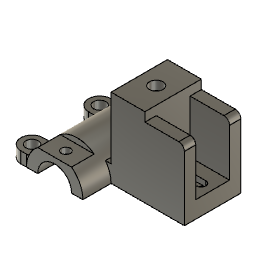
drawing_23 (Autodesk Fusion 360 design; units mm, degrees)
Autodesk Fusion 360 part; units mm, degrees
sketch "Sketch1" plane through (0, 0, 0) normal (0, 0, 1) x (1, 0, 0)
  line L0 (0, 0) -> (-32.5, 0)
  line L1 (-32.5, 0) -> (-32.5, 25)
  line L2 (-32.5, 25) -> (32.5, 25)
  line L3 (32.5, 25) -> (32.5, -25)
  line L4 (32.5, -25) -> (-32.5, -25)
  line L5 (-32.5, -25) -> (-32.5, 25)
  dimension "d1" = 32.5
  dimension "d2" = 25
  dimension "d3" = 65
  dimension "d4" = 50
  constraint coincident L0.start origin
  constraint horizontal L0
  constraint perpendicular L0 L1
  constraint horizontal L2
  constraint vertical L3
  constraint horizontal L4
  constraint vertical L5
  measures "d1" distance of L0.start L0.end
  measures "d2" distance of L0.end L1.end
  measures "d3" distance of L1.end L2.end
  measures "d4" distance of L1.end L4.end
extrude "Extrude1" add sketch "Sketch1" along normal blind 62 makes body 1
sketch "Sketch2" plane through (0, -25, 0) normal (0, -1, 0) x (1, 0, 0)
  line L0 (-32.5, 0) -> (32.5, 0)
  line L1 (32.5, 0) -> (32.5, 62)
  line L2 (32.5, 62) -> (-32.5, 62)
  line L3 (-32.5, 62) -> (-32.5, 0)
  line L4 (32.5, 57) -> (32.5, 36)
  line L5 (27.5, 62) -> (24, 62)
  arc A0 (32.5, 57) -> (27.5, 62) centre (27.5, 57) ccw
  dimension "d7" = 5
  constraint coincident L1 L4.end
  constraint perpendicular L2 L4
  constraint coincident L2 L5.end
  constraint perpendicular L1 L5
  constraint tangent L4 A0
  constraint tangent L5 A0
  measures "d7" radius of A0
extrude "Extrude2" cut sketch "Sketch2" against normal blind 63 contours L1 L2 A0 bodies 1
sketch "Sketch3" plane through (0, 0, 62) normal (0, 0, 1) x (-1, 0, 0)
  line L0 (-27.5, 25) -> (-27.5, -25)
  line L1 (-27.5, -25) -> (32.5, -25)
  line L2 (32.5, -25) -> (32.5, 25)
  line L3 (32.5, 25) -> (-27.5, 25)
  line L4 (-32.5, -25) -> (-27.5, -25)
  line L5 (-27.5, -25) -> (-27.5, 25)
  line L6 (-27.5, 25) -> (-32.5, 25)
  line L7 (-32.5, 25) -> (-32.5, -25)
  line L8 (-32.5, 0) -> (-32.5, -15)
  line L9 (-32.5, 0) -> (-32.5, 15)
  line L10 (-32.5, -15) -> (2.5, -15)
  line L11 (2.5, -15) -> (2.5, 15)
  line L12 (2.5, 15) -> (-32.5, 15)
  dimension "d10" = 15
  dimension "d11" = 15
  dimension "d12" = 35
  constraint midpoint L7 L8.start
  constraint perpendicular L1 L8
  constraint parallel L7 L9
  constraint perpendicular L7 L10
  constraint perpendicular L10 L11
  constraint perpendicular L9 L12
  measures "d10" distance of L8.start L8.end
  measures "d11" distance of L8.start L9.end
  measures "d12" distance of L8.end L10.end
extrude "Extrude3" cut sketch "Sketch3" against normal blind 47 contours L0 L5 L10 L11 L12 | L0 L5 L7 L8 L9 L10 L12 bodies 1
sketch "Sketch4" plane through (0, 0, 62) normal (0, 0, 1) x (-1, 0, 0)
  line L0 (2.5, -15) -> (-27.5, -15)
  line L1 (-27.5, -15) -> (-27.5, -25)
  line L2 (-27.5, -25) -> (32.5, -25)
  line L3 (32.5, -25) -> (32.5, 25)
  line L4 (32.5, 25) -> (-27.5, 25)
  line L5 (-27.5, 25) -> (-27.5, 15)
  line L6 (-27.5, 15) -> (2.5, 15)
  line L7 (2.5, 15) -> (2.5, -15)
  line L8 (32.5, -25) -> (2.5, -25)
  line L9 (2.5, -25) -> (2.5, 25)
  line L10 (2.5, 25) -> (32.5, 25)
  line L11 (32.5, 25) -> (32.5, -25)
  constraint horizontal L8
  constraint vertical L9
  constraint horizontal L10
  constraint vertical L11
  constraint midpoint L4 L9.end
  constraint coincident L2.end L3.start
extrude "Extrude4" add sketch "Sketch4" along normal blind 8 contours L2 L3 L4 L7 L8 L9 L10 L11 bodies 1
sketch "Sketch5" plane through (0, -25, 0) normal (0, -1, 0) x (1, 0, 0)
  arc A0 (32.5, 57) -> (27.5, 62) centre (27.5, 57) ccw
  line L0 (27.5, 62) -> (-2.5, 62)
  line L1 (-2.5, 62) -> (-2.5, 70)
  line L2 (-2.5, 70) -> (-32.5, 70)
  line L3 (-32.5, 70) -> (-32.5, 0)
  line L4 (-32.5, 0) -> (32.5, 0)
  line L5 (32.5, 0) -> (32.5, 57)
sketch "Sketch6" plane through (0, 0, 15) normal (0, 0, 1) x (-1, 0, 0)
  line L0 (-32.5, 15) -> (-32.5, -15)
  line L1 (-32.5, -15) -> (2.5, -15)
  line L2 (2.5, -15) -> (2.5, 15)
  line L3 (2.5, 15) -> (-32.5, 15)
  line L4 (32.5, 25) -> (2.5, 25)
  line L5 (2.5, 25) -> (2.5, -25)
  line L6 (2.5, -25) -> (32.5, -25)
  line L7 (32.5, -25) -> (32.5, 25)
  line L8 (17.5, 0) -> (-7.5, 0) construction
  line L9 (-7.5, 0) -> (-22.5, 0) construction
  line L10 (-7.5, 4) -> (-22.5, 4)
  arc A0 (-22.5, 4) -> (-22.5, -4) centre (-22.5, 0) ccw
  line L11 (-22.5, -4) -> (-7.5, -4)
  arc A1 (-7.5, -4) -> (-7.5, 4) centre (-7.5, 0) ccw
  line L12 (-7.5, 0) -> (-22.5, 0) construction
  point P0 (17.5, -25)
  point P1 (17.5, 0)
  point P2 (-15, -15)
  point P3 (-15, 0)
  dimension "d17" = 25
  dimension "d18" = 15
  dimension "d19" = 8
  constraint midpoint L6 P0
  constraint midpoint L1 P2
  constraint coincident P1 L8.start
  constraint perpendicular L2 L8
  constraint perpendicular L2 L9
  constraint tangent L10 A0
  constraint tangent A0 L11
  constraint parallel L10 L11
  constraint tangent L11 A1
  constraint tangent L10 A1
  constraint coincident L9.end A0.centre
  constraint perpendicular L0 L12
  constraint coincident L8.end L9.start
  measures "d17" distance of P1 L8.end
  measures "d18" distance of L8.end L9.end
  measures "d19" diameter of A0
extrude "Extrude5" cut sketch "Sketch6" against normal blind 5 contours L10 A0 L11 A1 bodies 1
sketch "Sketch7" plane through (0, 0, 10) normal (0, 0, 1) x (-1, 0, 0)
  arc A0 (-7.5, -4) -> (-7.5, 4) centre (-7.5, 0) ccw
  line L0 (-7.5, 4) -> (-22.5, 4)
  arc A1 (-22.5, 4) -> (-22.5, -4) centre (-22.5, 0) ccw
  line L1 (-22.5, -4) -> (-7.5, -4)
  circle A2 centre (-7.5, 0) radius 4
  circle A3 centre (-22.5, 0) radius 4
  dimension "d22" = 8
  dimension "d23" = 8
  constraint concentric A0 A2
  constraint concentric A1 A3
  measures "d22" diameter of A2
  measures "d23" diameter of A3
extrude "Extrude6" cut sketch "Sketch7" against normal blind 35 contours A0 A2 | A1 A3 bodies 1
sketch "Sketch8" plane through (0, 0, 70) normal (0, 0, 1) x (-1, 0, 0)
  line L0 (32.5, 25) -> (2.5, 25)
  line L1 (2.5, 25) -> (2.5, -25)
  line L2 (2.5, -25) -> (32.5, -25)
  line L3 (32.5, -25) -> (32.5, 25)
  circle A0 centre (17.5, 0) radius 6
  point P0 (17.5, -25)
  point P1 (17.5, 0)
  point P2 (17.5, 0)
  dimension "d26" = 12
  constraint midpoint L2 P0
  constraint coincident P2 P1
  measures "d26" diameter of A0
extrude "Extrude7" cut sketch "Sketch8" against normal blind 111 contours A0 bodies 1
sketch "Sketch9" plane through (0, 0, 0) normal (0, 0, -1) x (1, 0, 0)
  circle A0 centre (-17.5, 0) radius 6
  circle A1 centre (22.5, 0) radius 4
  circle A2 centre (7.5, 0) radius 4
  line L0 (32.5, 25) -> (-32.5, 25)
  line L1 (-32.5, 25) -> (-32.5, -25)
  line L2 (-32.5, -25) -> (32.5, -25)
  line L3 (32.5, -25) -> (32.5, 25)
  line L4 (-7.5, 15) -> (-27.5, 15)
  line L5 (-27.5, 15) -> (-27.5, -15)
  line L6 (-27.5, -15) -> (-7.5, -15)
  line L7 (-7.5, -15) -> (-7.5, 15)
  line L8 (-7.5, 15) -> (-27.5, -15) construction
  line L9 (-27.5, 15) -> (-7.5, -15) construction
  point P0 (-17.5, 0)
  dimension "d29" = 20
  dimension "d30" = 30
  constraint horizontal L4
  constraint perpendicular L4 L5
  constraint parallel L4 L6
  constraint parallel L5 L7
  constraint coincident L8 P0
  constraint coincident L9 P0
  constraint coincident P0 A0.centre
  measures "d29" distance of L5.end L6.end
  measures "d30" distance of L4.end L5.end
extrude "Extrude8" cut sketch "Sketch9" against normal blind 62 contours L4 L5 L6 L7 bodies 1
sketch "Sketch10" plane through (0, -25, 0) normal (0, -1, 0) x (1, 0, 0)
  line L0 (32.5, 0) -> (-57.5, 0) construction
  line L1 (-82.5, -0.0011) -> (-32.5, -0.0011) construction
  line L2 (-32.5, -0.0011) -> (-82.5, -0.0011)
  arc A0 (-32.5, -0.0011) -> (-82.5, -0.0011) centre (-57.5, 0) ccw
  dimension "d33" = 90
  dimension "d34" = 50
  constraint horizontal L0
  constraint coincident L0.end A0.centre
  constraint horizontal L1
  measures "d33" distance of L0.start L0.end
  measures "d34" diameter of A0
extrude "Extrude9" add sketch "Sketch10" against normal blind 55 separate body makes body 2
sketch "Sketch11" plane through (0, -25, 0) normal (0, -1, 0) x (1, 0, 0)
  arc A0 (-32.5, -0.0011) -> (-82.5, -0.0011) centre (-57.5, 0) ccw
  line L0 (-82.5, -0.0011) -> (-32.5, -0.0011)
  line L1 (-72.5, -0.0011) -> (-42.5, -0.0011)
  arc A1 (-42.5, -0.0011) -> (-72.5, -0.0011) centre (-57.5, 0) ccw
  dimension "d37" = 30
  constraint concentric A0 A1
  constraint coincident L0 L1.start
  constraint coincident L0 L1.end
  measures "d37" diameter of A1
extrude "Extrude10" cut sketch "Sketch11" against normal blind 30 contours L0 L1 A1 bodies 2
sketch "Sketch12" plane through (0, -25, 0) normal (0, -1, 0) x (1, 0, 0)
  arc A0 (-42.5, -0.0011) -> (-72.5, -0.0011) centre (-57.5, 0) ccw
  line L0 (-42.5, -0.0011) -> (-32.5, -0.0011)
  arc A1 (-32.5, -0.0011) -> (-82.5, -0.0011) centre (-57.5, 0) ccw
  line L1 (-82.5, -0.0011) -> (-72.5, -0.0011)
  circle A2 centre (-57.5, 0) radius 5
  circle A3 centre (-57.5, 0) radius 10
  dimension "d40" = 10
  dimension "d41" = 20
  constraint concentric A0 A2
  constraint concentric A0 A3
  measures "d40" diameter of A2
  measures "d41" diameter of A3
extrude "Extrude11" cut sketch "Sketch12" against normal blind 90 contours A2 | A3 bodies 2
sketch "Sketch13" plane through (0, -25, 0) normal (0, -1, 0) x (1, 0, 0)
  arc A0 (-42.5, -0.0011) -> (-72.5, -0.0011) centre (-57.5, 0) ccw
  line L0 (-42.5, -0.0011) -> (-32.5, -0.0011)
  arc A1 (-32.5, -0.0011) -> (-82.5, -0.0011) centre (-57.5, 0) ccw
  line L1 (-82.5, -0.0011) -> (-72.5, -0.0011)
  line L2 (-57.5, 0) -> (-57.5, 20) construction
  line L3 (-42.5, 20) -> (-76.9384, 20)
  line L4 (-76.9384, 20) -> (-76.9384, 30.4087)
  line L5 (-76.9384, 30.4087) -> (-42.5, 30.4087)
  line L6 (-42.5, 30.4087) -> (-42.5, 20)
  dimension "d44" = 20
  constraint coincident A0.centre A1.centre
  constraint perpendicular L0 L2
  constraint horizontal L3
  constraint vertical L4
  constraint horizontal L5
  constraint vertical L6
  constraint coincident A1 L3.start
  measures "d44" distance of A0.centre L2.end
extrude "Extrude12" cut sketch "Sketch13" against normal blind 20 contours A1 L3 bodies 2
sketch "Sketch14" plane through (0, 30, 0) normal (0, 1, 0) x (-1, 0, 0)
  arc A0 (67.5, -0.0011) -> (47.5, -0.0011) centre (57.5, 0) ccw
  line L0 (67.5, -0.0011) -> (82.5, -0.0011)
  arc A1 (82.5, -0.0011) -> (32.5, -0.0011) centre (57.5, 0) ccw
  line L1 (32.5, -0.0011) -> (47.5, -0.0011)
extrude "Extrude13" add sketch "Sketch14" against normal blind 80 bodies 2 1
sketch "Sketch15" plane through (0, -50, 0) normal (0, -1, 0) x (1, 0, 0)
  line L0 (-82.5, -0.0011) -> (-67.5, -0.0011)
  arc A0 (-47.5, -0.0011) -> (-67.5, -0.0011) centre (-57.5, 0) ccw
  line L1 (-47.5, -0.0011) -> (-32.5, -0.0011)
  arc A1 (-32.5, -0.0011) -> (-82.5, -0.0011) centre (-57.5, 0) ccw
  circle A2 centre (-57.5, 0) radius 15
  dimension "d49" = 30
  constraint concentric A0 A2
  measures "d49" diameter of A2
extrude "Extrude14" cut sketch "Sketch15" against normal blind 30 contours L0 A0 L1 A2 picked at (-44.2597, 1.2413) bodies 2
sketch "Sketch16" plane through (0, -50, 0) normal (0, -1, 0) x (1, 0, 0)
  arc A0 (-42.5, -0.0011) -> (-72.5, -0.0011) centre (-57.5, 0) ccw
  line L0 (-42.5, -0.0011) -> (-32.5, -0.0011)
  arc A1 (-32.5, -0.0011) -> (-82.5, -0.0011) centre (-57.5, 0) ccw
  line L1 (-82.5, -0.0011) -> (-72.5, -0.0011)
  line L2 (-57.5, 0) -> (-57.5, 20) construction
  line L3 (-42.5, 20) -> (-77.6563, 20)
  line L4 (-77.6563, 20) -> (-77.6563, 34.6446)
  line L5 (-77.6563, 34.6446) -> (-42.5, 34.6446)
  line L6 (-42.5, 34.6446) -> (-42.5, 20)
  constraint coincident A0.centre A1.centre
  constraint vertical L2
  constraint horizontal L3
  constraint vertical L4
  constraint horizontal L5
  constraint vertical L6
  constraint coincident A1 L3.start
extrude "Extrude15" cut sketch "Sketch16" against normal blind 20 contours A1 L3 bodies 2
sketch "Sketch17" plane through (0, 0, 20) normal (0, 0, 1) x (-1, 0, 0)
  line L0 (72.5, 50) -> (42.5, 50)
  line L1 (42.5, 50) -> (42.5, 30)
  line L2 (42.5, 30) -> (72.5, 30)
  line L3 (72.5, 30) -> (72.5, 50)
  circle A0 centre (57.5, 40) radius 4
  dimension "d54" = 8
  measures "d54" diameter of A0
extrude "Extrude16" cut sketch "Sketch17" against normal blind 40 contours A0 bodies 2
sketch "Sketch18" plane through (0, -25, 35) normal (0, -1, 0) x (1, 0, 0)
sketch "Sketch19" plane through (-32.5, 0, 0) normal (-1, 0, 0) x (0, -1, 0)
  line L0 (-25, 0) -> (25, 0)
  line L1 (25, 0) -> (25, 70)
  line L2 (25, 70) -> (-25, 70)
  line L3 (-25, 70) -> (-25, 0)
  line L4 (25, 0) -> (25, 15) construction
  line L5 (25, 15) -> (-25, 15)
  line L6 (-25, 15) -> (-25, 0)
  line L7 (-25, 0) -> (25, 0)
  line L8 (25, 0) -> (25, 15)
  constraint coincident L0.end L1.start
  constraint coincident L1 L4.end
  constraint perpendicular L0 L4
  constraint horizontal L5
  constraint vertical L6
  constraint horizontal L7
  constraint vertical L8
  constraint coincident L0.start L3.end
extrude "Extrude17" add sketch "Sketch19" along normal blind 9 contours L0 L1 L3 L5 L6 L7 L8 bodies 2
sketch "Sketch20" plane through (0, 0, 0) normal (0, 0, 1) x (1, 0, 0)
  line L0 (-72.5, -50) -> (-72.5, -30)
  line L1 (-42.5, -30) -> (-72.5, -30)
  line L2 (-42.5, -30) -> (-42.5, -50)
  line L3 (-42.5, -50) -> (-32.5, -50)
  line L4 (-32.5, -50) -> (-32.5, 30)
  line L5 (-32.5, 30) -> (-82.5, 30)
  line L6 (-82.5, 30) -> (-82.5, -50)
  line L7 (-82.5, -50) -> (-72.5, -50)
  line L8 (-37.5, -25) -> (-32.5, -25)
  line L9 (-37.5, -25) -> (-37.5, 25)
  line L10 (-32.5, 25) -> (-37.5, 25)
  line L11 (-32.5, 25) -> (-32.5, -25)
  line L12 (-82.5, -10) -> (-82.5, 20) construction
  line L13 (-82.5, -10) -> (-82.5, -40) construction
  line L14 (-67.5, -20) -> (-47.5, -20) construction
  line L15 (-67.5, -20) -> (-67.5, 30) construction
  line L16 (-67.5, 30) -> (-47.5, 30) construction
  line L17 (-47.5, 30) -> (-47.5, -20) construction
  line L18 (-57.5, 30) -> (-87.5, 30) construction
  line L19 (-87.5, 30) -> (-87.5, -50) construction
  circle A0 centre (-87.5, 20) radius 10
  circle A1 centre (-87.5, -39.9992) radius 10
  line L20 (-87.5, 30) -> (-82.5, 30)
  line L21 (-87.5, 10) -> (-82.5, 10)
  line L22 (-87.5, -29.9992) -> (-82.5, -29.9992)
  point P0 (-82.5, -10)
  point P1 (-57.5, 30)
  point P2 (-87.5, -39.9992)
  point P3 (-87.5, 20)
  dimension "d60" = 30
  dimension "d61" = 30
  dimension "d62" = 30
  dimension "d63" = 20
  dimension "d64" = 20
  dimension "d65" = 180
  constraint midpoint L6 P0
  constraint coincident P0 L12.start
  constraint parallel L6 L12
  constraint parallel L6 L13
  constraint midpoint L16 P1
  constraint coincident P1 L18.start
  constraint parallel L16 L18
  constraint perpendicular L7 L19
  constraint coincident L19 P2
  constraint coincident L19 P3
  constraint coincident P3 A0.centre
  constraint coincident P2 A1.centre
  constraint coincident L5.end L6.start
  constraint coincident A0 L21.start
  constraint coincident L19 L21.start
  constraint coincident L12 L21.end
  constraint coincident L19 L22.start
  constraint coincident A1 L22.start
  constraint perpendicular L13 L22
  measures "d60" distance of P0 L12.end
  measures "d61" distance of P0 L13.end
  measures "d62" distance of P1 L18.end
  measures "d63" diameter of A0
  measures "d64" diameter of A1
  measures "d65" angle of L21 L22
sketch "Sketch22" plane through (0, 0, 0) normal (0, 0, 1) x (1, 0, 0)
sketch "Sketch21" plane through (0, 0, 0) normal (0, 0, 1) x (1, 0, 0)
  line L0 (-87.5, -50) -> (-82.5, -50)
  line L1 (-87.5, -30) -> (-82.5, -30)
  arc A0 (-87.5, -30) -> (-87.5, -50) centre (-87.5, -40) ccw
  line L2 (-82.5, -50) -> (-82.5, -30)
  line L3 (-82.5, -30) -> (-82.5, 30)
  dimension "d66" = 20
  constraint horizontal L0
  constraint tangent L1 A0
  constraint horizontal L1
  constraint perpendicular L1 L3
  measures "d66" diameter of A0
extrude "Extrude18" add sketch "Sketch21" sketch "Sketch20" along normal blind 10 separate body of sketch 2 contours L6 A1 | L6 A1 L22 | L6 A0 L21 | L6 A0 | L6 A0 L20 picked at (-87.8349, -39.3827) picked at (-90.1061, 22.0783) makes body 3 at (-89.4815, 10.1983, 6.6667) makes body 4 at (-90.8333, -40.0106, 0)
extrude "Extrude19" add 1 faces at (-82.5, 23.3333, 3.3333) along direction (1, 0, 0) blind 5 on bodies 3 bodies 3 4 2
extrude "Extrude20" add 2 faces at (-82.5, -43.3333, 3.3333) (-82.5, -29.9995, 3.3333) along direction (1, 0, 0) blind 5 on bodies 4 bodies 4 3
sketch "Sketch23" plane through (0, 0, 10) normal (0, 0, 1) x (-1, 0, 0)
  arc A0 (87.4986, -30) -> (87.5, -10) centre (87.5, -20) ccw
  line L0 (87.5, -10) -> (80.4129, -10)
  line L1 (80.4129, -10) -> (80.4129, -30)
  line L2 (80.4129, -30) -> (82.5, -30)
  line L3 (82.5, -30) -> (87.4986, -30)
  circle A1 centre (87.5, -20) radius 10
  constraint concentric A0 A1
  constraint coincident A0.start A1
extrude "Extrude21" cut sketch "Sketch23" along normal blind 6 contours A0 L1 A1 | L1 A1 bodies 4
sketch "Sketch24" plane through (0, 0, 10) normal (0, 0, 1) x (-1, 0, 0)
  arc A0 (97.4999, 40.0327) -> (87.5, 50) centre (87.5, 40) ccw
  line L0 (87.5, 50) -> (82.5, 50)
  line L1 (82.5, 50) -> (80.4129, 50)
  line L2 (80.4129, 50) -> (80.4129, 30)
  line L3 (80.4129, 30) -> (82.5, 30)
  line L4 (82.5, 30) -> (82.5, 29.9992)
  line L5 (82.5, 29.9992) -> (87.5, 29.9992)
  arc A1 (87.5, 29.9992) -> (97.4999, 40.0327) centre (87.5, 39.9992) ccw
  circle A2 centre (87.5, 39.9992) radius 10
  constraint concentric A1 A2
  constraint coincident L5.end A2
extrude "Extrude22" cut sketch "Sketch24" along normal blind 31 contours L2 A1 A2 | L2 A2 bodies 4
sketch "Sketch25" plane through (0, 0, 0) normal (0, 0, 1) x (1, 0, 0)
  arc A0 (-87.4986, 30) -> (-87.5, 10) centre (-87.5, 20) ccw
  line L0 (-87.4986, 30) -> (-82.5, 30)
  line L1 (-82.5, 30) -> (-82.5, 10)
  line L2 (-82.5, 10) -> (-87.5, 10)
  line L3 (-82.5, -30) -> (-82.5, -50)
  line L4 (-82.5, -50) -> (-87.5, -50)
  arc A1 (-97.4999, -40.0327) -> (-87.5, -50) centre (-87.5, -40) ccw
  arc A2 (-87.5, -29.9992) -> (-97.4999, -40.0327) centre (-87.5, -39.9992) ccw
  line L5 (-87.5, -29.9992) -> (-82.5, -29.9992)
  line L6 (-82.5, -29.9992) -> (-82.5, -30)
  circle A3 centre (-87.5, 20) radius 5.5
  circle A4 centre (-87.5, -40) radius 5.5
  dimension "d77" = 11
  dimension "d78" = 11
  constraint concentric A0 A3
  constraint concentric A1 A4
  measures "d77" diameter of A3
  measures "d78" diameter of A4
extrude "Extrude23" cut sketch "Sketch25" along normal blind 16 contours L1 A3 | L1 A3 | L3 A4 | L3 A4 bodies 4
equation "d1 = ( 65 / 2 ) * 1 mm"
equation "d13 = -62 mm + 15 mm"
